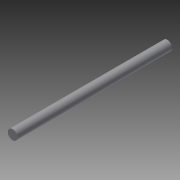
# Autodesk Inventor part: rod
Saved by Autodesk Inventor 2014 (Build 180170000, 170)
## iProperties
Created: 2014-05-19
Part Number: rod
Material: Generic
Document SubType Name: Modeling
Designer: jyesowitz
Density: 1 g/cm^3
Appearance: Default
Author: jyesowitz
Autodesk Inventor part; units mm, degrees
ref_plane "YZ Plane" through (0, 0, 0) normal (1, 0, 0) x (0, 1, 0)
ref_plane "XZ Plane" through (0, 0, 0) normal (0, 1, 0) x (-1, 0, 0)
ref_plane "XY Plane" through (0, 0, 0) normal (0, 0, 1) x (1, 0, 0)
sketch "Sketch1" plane through (0, 0, 0) normal (0, 0, 1) x (1, 0, 0)
  circle A0 centre (0, 0) radius 6.35
  dimension "d0" = 12.7
  constraints: 1 centre point, 1 coincident
  measures "d0" diameter of A0
extrude "Extrusion1" add sketch "Sketch1" against normal blind 203.2
body "Solid1"
